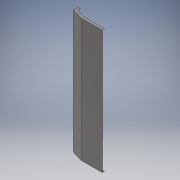
# Autodesk Inventor part: Cover Lower Front
Saved by Autodesk Inventor 2018 (Build 220112000, 112)
## iProperties
Created: 2018-08-07
Part Number: Cover Lower Front
Material: Steel
Document SubType Name: Modeling
Designer: P301319
Density: 7.85 g/cm^3
Appearance: Stainless - Brushed
Author: P301319
Autodesk Inventor part; units mm, degrees
ref_plane "YZ Plane" through (0, 0, 0) normal (1, 0, 0) x (0, 1, 0)
ref_plane "XZ Plane" through (0, 0, 0) normal (0, 1, 0) x (-1, 0, 0)
ref_plane "XY Plane" through (0, 0, 0) normal (0, 0, 1) x (1, 0, 0)
sketch "Sketch1" plane through (0, 0, 0) normal (0, 0, 1) x (1, 0, 0)
  line L0 (0, 0) -> (200, 0)
  line L1 (0, 0) -> (-100, 30)
  line L2 (0, 0) -> (104.4031, 0) construction
  line L3 (-100, 30) -> (-100, 69)
  line L4 (-98.4, 69) -> (-98.4, 31.1904)
  line L5 (-98.4, 31.1904) -> (0.2348, 1.6)
  line L6 (0.2348, 1.6) -> (200, 1.6)
  line L7 (-98.4, 69) -> (-100, 69)
  line L8 (200, 1.6) -> (200, 0)
  dimension "d0" = 200
  dimension "d2" = 100
  dimension "d3" = 39
  dimension "d9" = 30
  dimension "d10" = 1.6
  constraints: 18 end point, 3 horizontal, 2 vertical, 1 equal length, 2 other
  measures "d0" distance of L0.start L0.end
  measures "d2" horizontal distance of L0.start L1.end
  measures "d3" distance of L1.end L3.end
  measures "d9" vertical distance of L0.start L1.end
  measures "d10" distance between parallel lines of L1 L5
extrude "Extrusion1" add sketch "Sketch1" along normal blind 1160
sketch "Sketch2" plane through (0, 0, 1160) normal (0, 0, 1) x (1, 0, 0)
  line L0 (-98.4, 31.1904) -> (-98.4, 69) projected
  line L1 (0.2348, 1.6) -> (-98.4, 31.1904) projected
  line L2 (200, 1.6) -> (0.2348, 1.6) projected
  line L3 (-78.4, 69) -> (-78.4, 46.0711)
  line L4 (-78.4, 46.0711) -> (3.1702, 21.6)
  line L5 (3.1702, 21.6) -> (200, 21.6)
  line L6 (-78.4, 69) -> (-98.4, 69)
  line L7 (200, 21.6) -> (200, 1.6)
  point P0 (0, 0)
  dimension "d11" = 20
  constraints: 10 end point, 1 horizontal, 1 vertical, 2 other
  measures "d11" distance between parallel lines of L1 L4
extrude "Extrusion2" add sketch "Sketch2" against normal blind 1.6
sketch "Sketch3" plane through (0, 0, 0) normal (0, 0, -1) x (-1, 0, 0)
  line L0 (98.4, 69) -> (98.4, 31.1904) projected
  line L1 (98.4, 69) -> (78.4, 69) projected
  line L2 (78.4, 69) -> (78.4, 46.0711) projected
  line L3 (78.4, 46.0711) -> (-3.1702, 21.6) projected
  line L4 (-3.1702, 21.6) -> (-200, 21.6) projected
  line L5 (-200, 21.6) -> (-200, 1.6) projected
  line L6 (-0.2348, 1.6) -> (-200, 1.6) projected
  line L7 (98.4, 31.1904) -> (-0.2348, 1.6) projected
  point P0 (0, 0)
extrude "Extrusion3" add sketch "Sketch3" against normal blind 1.6
body "Solid1"
